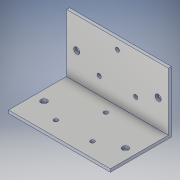
# Autodesk Inventor part: bracket_design2
Saved by Autodesk Inventor 2017 (Build 210142000, 142)
## iProperties
Created: 2018-04-04
Part Number: bracket_design2
Material: Aluminum 6061
Document SubType Name: Modeling
Designer: Roland
Density: 2.7 g/cm^3
Appearance: Aluminum - Flat
Author: Roland
Autodesk Inventor part; units mm, degrees
ref_plane "YZ Plane" through (0, 0, 0) normal (1, 0, 0) x (0, 1, 0)
ref_plane "XZ Plane" through (0, 0, 0) normal (0, 1, 0) x (-1, 0, 0)
ref_plane "XY Plane" through (0, 0, 0) normal (0, 0, 1) x (1, 0, 0)
sketch "Sketch7" plane through (0, 0, 0) normal (0, 0, 1) x (1, 0, 0)
  line L0 (25, -15) -> (-25, -15)
  line L1 (-25, -15) -> (-25, 15)
  line L2 (-25, 15) -> (25, 15)
  line L3 (25, 15) -> (25, -15)
  line L4 (25, -15) -> (-25, 15) construction
  line L5 (-25, -15) -> (25, 15) construction
  point P0 (0, 0)
  dimension "d37" = 50
  dimension "d38" = 30
  constraints: 12 end point, 2 midpoint, 2 parallel, 1 horizontal, 1 perpendicular
  measures "d37" distance of L1.end L2.end
  measures "d38" distance of L0.end L1.end
extrude "Extrusion4" add sketch "Sketch7" along normal blind 1.5
sketch "Sketch8" plane through (0, 0, 1.5) normal (0, 0, 1) x (1, 0, 0)
  line L0 (-25, -15) -> (25, -15) projected
  line L1 (-25, 15) -> (-25, -15) projected
  line L2 (25, -15) -> (-25, -15)
  line L3 (-25, -15) -> (-25, -13.5)
  line L4 (-25, -13.5) -> (25, -13.5)
  line L5 (25, -13.5) -> (25, -15)
  point P0 (0, 0)
  dimension "d41" = 1.5
  constraints: 8 end point, 2 parallel, 1 horizontal, 1 perpendicular, 1 point on line
  measures "d41" distance of L2.end L3.end
extrude "Extrusion5" add sketch "Sketch8" along normal blind 28.5
sketch "Sketch14" plane through (0, 0, 0) normal (0, 0, -1) x (-1, 0, 0)
  circle A0 centre (0, 0) radius 8.5
  line L0 (-1.5, 8.3666) -> (-1.5, 10.3666)
  line L1 (-1.5, 8.3666) -> (0.5, 8.3666) construction
  line L2 (1.5, 8.3666) -> (1.5, 10.3666)
  arc A1 (1.5, 10.3666) -> (-1.5, 10.3666) centre (0, 10.3666) ccw
  line L3 (-6.4957, -5.4823) -> (-8.2277, -6.4823)
  arc A2 (-9.7277, -3.8843) -> (-8.2277, -6.4823) centre (-8.9777, -5.1833) ccw
  line L4 (-7.9957, -2.8843) -> (-9.7277, -3.8843)
  line L5 (7.9957, -2.8843) -> (9.7277, -3.8843)
  arc A3 (8.2277, -6.4823) -> (9.7277, -3.8843) centre (8.9777, -5.1833) ccw
  line L6 (6.4957, -5.4823) -> (8.2277, -6.4823)
  line L7 (-25, 15) -> (-25, -15) projected
  line L8 (25, -15) -> (25, 15) projected
  point P0 (-20, 0)
  point P1 (20, 0)
  dimension "d80" = 17
  dimension "d127" = 2
  dimension "d128" = 90
  dimension "d131" = 360
  dimension "d146" = 5
  dimension "d147" = 5
  constraints: 14 end point, 8 point on circle, 6 coincident, 4 centre point, 2 tangent, 2 vertical, 1 horizontal, 1 perpendicular, 29 other
  measures "d80" diameter of A0
  measures "d127" distance of L0.start L0.end
  measures "d128" angle of L1 L0
  measures "d146" distance from line of L7 point (-20, 0)
  measures "d147" distance from line of point (20, 0) L8
hole "Hole5" at (0, 10.3666, 0) at (-8.9777, -5.1833, 0) at (8.9777, -5.1833, 0) direction (0, 0, 1) diameter 2 end through all
hole "Hole6" at (-20, 0, 0) at (20, 0, 0) direction (0, 0, 1) diameter 3 end through all
sketch "Sketch17" plane through (0, -15, 17.5917) normal (0, -1, 0) x (-1, 0, 0)
  circle A0 centre (0, 0) radius 8.5
  line L0 (-1.5, 8.3666) -> (-1.5, 10.3666)
  line L1 (-1.5, 8.3666) -> (0.5, 8.3666) construction
  line L2 (1.5, 8.3666) -> (1.5, 10.3666)
  arc A1 (1.5, 10.3666) -> (-1.5, 10.3666) centre (0, 10.3666) ccw
  line L3 (-6.4957, -5.4823) -> (-8.2277, -6.4823)
  arc A2 (-9.7277, -3.8843) -> (-8.2277, -6.4823) centre (-8.9777, -5.1833) ccw
  line L4 (-7.9957, -2.8843) -> (-9.7277, -3.8843)
  line L5 (7.9957, -2.8843) -> (9.7277, -3.8843)
  arc A3 (8.2277, -6.4823) -> (9.7277, -3.8843) centre (8.9777, -5.1833) ccw
  line L6 (6.4957, -5.4823) -> (8.2277, -6.4823)
  line L7 (-25, 15) -> (-25, -15)
  line L8 (25, -15) -> (25, 15)
  point P0 (-20, 0)
  point P1 (20, 0)
  dimension "d155" = 17
  dimension "d154" = 2
  dimension "d169" = 90
  dimension "d151" = 360
  dimension "d153" = 5
  dimension "d152" = 5
  constraints: 18 end point, 8 point on circle, 6 coincident, 4 centre point, 2 tangent, 2 vertical, 1 horizontal, 1 perpendicular, 29 other
  measures "d155" diameter of A0
  measures "d154" distance of L0.start L0.end
  measures "d169" angle of L1 L0
  measures "d153" distance from line of L7 point (-20, 0)
  measures "d152" distance from line of point (20, 0) L8
hole "Hole10" at (0, -15, 7.225) at (-8.9777, -15, 22.775) at (8.9777, -15, 22.775) direction (0, 1, 0) diameter 2 end through all
hole "Hole11" at (-20, -15, 17.5917) at (20, -15, 17.5917) direction (0, 1, 0) diameter 3 end through all
body "Solid2"
